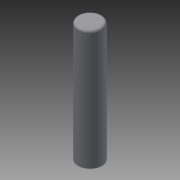
# Autodesk Inventor part: queue
Saved by Autodesk Inventor 2014 SP2 (Build 180246200, 246)
## iProperties
Created: 2015-03-17
Part Number: queue
Material: Générique
Document SubType Name: Modeling
Designer: sd
Density: 1 g/cm^3
Appearance: Par défaut
Mass: 0.00392055 g
Surface Area: 0.171395 cm^2
Volume: 0.00392055 cm^3
Author: sd
Autodesk Inventor part; units mm, degrees
ref_plane "YZ Plane" through (0, 0, 0) normal (1, 0, 0) x (0, 1, 0)
ref_plane "XZ Plane" through (0, 0, 0) normal (0, 1, 0) x (-1, 0, 0)
ref_plane "XY Plane" through (0, 0, 0) normal (0, 0, 1) x (1, 0, 0)
sketch "Esquisse1" plane through (0, 0, 0) normal (0, 0, 1) x (1, 0, 0)
  circle A0 centre (0, 0) radius 0.5
  dimension "d0" = 1
  constraints: 1 centre point, 1 coincident
  measures "d0" diameter of A0
extrude "Extrusion1" add sketch "Esquisse1" along normal blind 5
fillet "Congé1" radius 0.1 1 edges at (-0.5, 0, 5)
